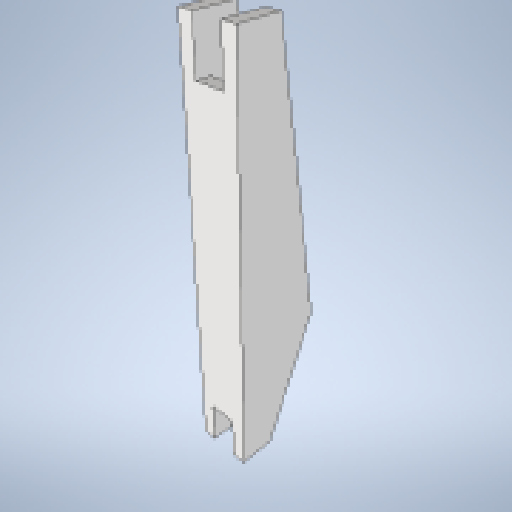
# Autodesk Inventor part: UpperArmBoundingBox
Saved by Autodesk Inventor 2023 (Build 270158000, 158)
## iProperties
Created: 2023-03-18
Part Number: UpperArmBoundingBox
Material: Generic
Document SubType Name: Modeling
Designer: Val
Density: 1 g/cm^3
Appearance: Default
Author: Val
Autodesk Inventor part; units mm, degrees
ref_plane "YZ Plane" through (0, 0, 0) normal (1, 0, 0) x (0, 1, 0)
ref_plane "XZ Plane" through (0, 0, 0) normal (0, 1, 0) x (-1, 0, 0)
ref_plane "XY Plane" through (0, 0, 0) normal (0, 0, 1) x (1, 0, 0)
sketch "BoundingBox" plane through (0, 0, 0) normal (1, 0, 0) x (0, 1, 0)
  line L0 (434.8115, 24.0504) -> (-18, 24.0504)
  line L1 (-18, 24.0504) -> (-18, -15.6719)
  line L2 (-18, -15.6719) -> (130.2861, -72.3729)
  line L3 (130.2861, -72.3729) -> (434.8115, -19.2646)
  line L4 (434.8115, -19.2646) -> (434.8115, 24.0504)
  point P0 (0, 0)
  point P1 (417.3115, 0.6447)
  point P2 (-18, 4.1892)
  dimension "d5" = 24.0504
  dimension "d6" = 4.1893
  dimension "d7" = 110.926
  dimension "d8" = 452.8115
  dimension "d9" = 39.7223
  dimension "d10" = 43.315
  dimension "d11" = 99.893
  dimension "d12" = 56.7009
  dimension "d13" = 17.5
  dimension "d14" = 23.4057
  constraints: 10 end point, 2 perpendicular, 1 midpoint
  measures "d5" distance from line of L0 point (0, 0)
  measures "d6" vertical distance of point (-18, 4.189) point (0, 0)
  measures "d7" angle of L1 L2
  measures "d8" distance of L0.start L0.end
  measures "d9" distance of L0.end L1.end
  measures "d10" distance of L3.end L0.start
  measures "d11" angle of L4 L3
  measures "d12" vertical distance of L1.end L2.end
  measures "d13" distance from line of L4 point (417.312, 0.645)
  measures "d14" distance from line of L0 point (417.312, 0.645)
extrude "BoundingBoxFeature" add sketch "BoundingBox" along normal mid plane 60
sketch "ForearmSpace" plane through (0, 0, 0) normal (0, 0, 1) x (1, 0, 0)
  line L0 (15, 142.9861) -> (-15, 142.9861)
  line L1 (-15, 142.9861) -> (-15, 434.8115)
  line L2 (-15, 434.8115) -> (15, 434.8115)
  line L3 (15, 434.8115) -> (15, 142.9861)
  line L4 (-30, 434.8115) -> (30, 434.8115) projected
  line L5 (0, -86.9623) -> (0, 521.7738) projected
  line L6 (30, 130.2861) -> (30, 434.8115) projected
  line L7 (-30, 130.2861) -> (30, 130.2861) projected
  line L8 (-30, 434.8115) -> (-30, 130.2861) projected
  line L9 (15, 142.9861) -> (-15, 142.9861)
  line L10 (-15, 142.9861) -> (-15, -18)
  line L11 (-15, -18) -> (15, -18)
  line L12 (15, -18) -> (15, 142.9861)
  line L13 (-30, -18) -> (30, -18) projected
  point P0 (0, 0)
  point P1 (-30, 282.5488)
  point P2 (0, 142.9861)
  dimension "d19" = 12.7
  dimension "d21" = 30
  constraints: 16 end point, 4 parallel, 3 collinear, 2 horizontal, 2 midpoint, 2 perpendicular, 1 point on line
  measures "d19" distance between parallel lines of L7 L0
  measures "d21" distance between parallel lines of L1 L3
extrude "ForearmCutFeature" cut sketch "ForearmSpace" along normal through all both and the other way through all contours L12 L7 L5 L0 | L0 L5 L2 L3 | L5 L7 L10 L0 | L0 L1 L2 L5 | L12 L11 L5 L7 | L5 L11 L10 L7
sketch "Sketch4" plane through (30, 0, 0) normal (1, 0, 0) x (0, 0, -1)
  line L0 (-24.0504, 434.8115) -> (-24.0504, -18) projected
  line L1 (-24.0504, 32.8) -> (-9.0504, 32.8)
  line L2 (-9.0504, 32.8) -> (-9.0504, 384.0115)
  line L3 (-9.0504, 384.0115) -> (-24.0504, 384.0115)
  line L4 (-24.0504, 384.0115) -> (-24.0504, 32.8)
  line L5 (-24.0504, -18) -> (15.6719, -18) projected
  line L6 (19.2646, 434.8115) -> (-24.0504, 434.8115) projected
  point P0 (0, 0)
  dimension "d25" = 15
  dimension "d26" = 50.8
  dimension "d27" = 50.8
  constraints: 8 end point, 2 parallel, 1 horizontal, 1 perpendicular, 1 point on line
  measures "d25" distance of L1.start L1.end
  measures "d26" distance between parallel lines of L5 L1
  measures "d27" distance between parallel lines of L6 L3
extrude "Extrusion3" add sketch "Sketch4" against normal up to surface (45 mm away)
body "Solid1"
